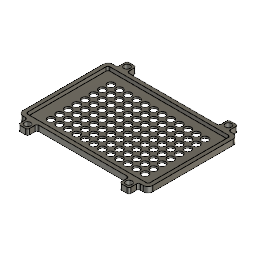
Plate_Adaptor_96 (Autodesk Fusion 360 design; units mm, degrees)
Autodesk Fusion 360 part; units mm, degrees
sketch "Sketch1" plane through (0, 0, 0) normal (0, 0, 1) x (1, 0, 0)
  line L0 (-68.38, 47.37) -> (68.38, 47.37)
  line L1 (68.38, 47.37) -> (68.38, -47.37)
  line L2 (68.38, -47.37) -> (-68.38, -47.37)
  line L3 (-68.38, -47.37) -> (-68.38, 47.37)
  line L4 (-68.38, 47.37) -> (68.38, -47.37) construction
  line L5 (68.38, 47.37) -> (-68.38, -47.37) construction
  line L6 (-58.38, 57.37) -> (-48.38, 57.37)
  line L7 (-48.38, 57.37) -> (-48.38, 47.37)
  line L8 (-48.38, 47.37) -> (-58.38, 47.37)
  line L9 (-58.38, 47.37) -> (-58.38, 57.37)
  line L10 (48.38, 57.37) -> (58.38, 57.37)
  line L11 (58.38, 57.37) -> (58.38, 47.37)
  line L12 (58.38, 47.37) -> (48.38, 47.37)
  line L13 (48.38, 47.37) -> (48.38, 57.37)
  line L14 (48.38, -47.37) -> (58.38, -47.37)
  line L15 (58.38, -47.37) -> (58.38, -57.37)
  line L16 (58.38, -57.37) -> (48.38, -57.37)
  line L17 (48.38, -57.37) -> (48.38, -47.37)
  line L18 (-58.38, -47.37) -> (-48.38, -47.37)
  line L19 (-48.38, -47.37) -> (-48.38, -57.37)
  line L20 (-48.38, -57.37) -> (-58.38, -57.37)
  line L21 (-58.38, -57.37) -> (-58.38, -47.37)
  line L22 (-49.5, 31.5) -> (49.5, 31.5)
  line L23 (49.5, 31.5) -> (49.5, -31.5)
  line L24 (49.5, -31.5) -> (-49.5, -31.5)
  line L25 (-49.5, -31.5) -> (-49.5, 31.5)
  line L26 (-49.5, 31.5) -> (49.5, -31.5) construction
  line L27 (49.5, 31.5) -> (-49.5, -31.5) construction
  circle A0 centre (-49.5, -31.5) radius 3.575
  circle A1 centre (-40.5, -31.5) radius 3.575
  circle A2 centre (-31.5, -31.5) radius 3.575
  circle A3 centre (-22.5, -31.5) radius 3.575
  circle A4 centre (-13.5, -31.5) radius 3.575
  circle A5 centre (-4.5, -31.5) radius 3.575
  circle A6 centre (4.5, -31.5) radius 3.575
  circle A7 centre (13.5, -31.5) radius 3.575
  circle A8 centre (22.5, -31.5) radius 3.575
  circle A9 centre (31.5, -31.5) radius 3.575
  circle A10 centre (40.5, -31.5) radius 3.575
  circle A11 centre (49.5, -31.5) radius 3.575
  circle A12 centre (-49.5, -22.5) radius 3.575
  circle A13 centre (-40.5, -22.5) radius 3.575
  circle A14 centre (-31.5, -22.5) radius 3.575
  circle A15 centre (-22.5, -22.5) radius 3.575
  circle A16 centre (-13.5, -22.5) radius 3.575
  circle A17 centre (-4.5, -22.5) radius 3.575
  circle A18 centre (4.5, -22.5) radius 3.575
  circle A19 centre (13.5, -22.5) radius 3.575
  circle A20 centre (22.5, -22.5) radius 3.575
  circle A21 centre (31.5, -22.5) radius 3.575
  circle A22 centre (40.5, -22.5) radius 3.575
  circle A23 centre (49.5, -22.5) radius 3.575
  circle A24 centre (-49.5, -13.5) radius 3.575
  circle A25 centre (-40.5, -13.5) radius 3.575
  circle A26 centre (-31.5, -13.5) radius 3.575
  circle A27 centre (-22.5, -13.5) radius 3.575
  circle A28 centre (-13.5, -13.5) radius 3.575
  circle A29 centre (-4.5, -13.5) radius 3.575
  circle A30 centre (4.5, -13.5) radius 3.575
  circle A31 centre (13.5, -13.5) radius 3.575
  circle A32 centre (22.5, -13.5) radius 3.575
  circle A33 centre (31.5, -13.5) radius 3.575
  circle A34 centre (40.5, -13.5) radius 3.575
  circle A35 centre (49.5, -13.5) radius 3.575
  circle A36 centre (-49.5, -4.5) radius 3.575
  circle A37 centre (-40.5, -4.5) radius 3.575
  circle A38 centre (-31.5, -4.5) radius 3.575
  circle A39 centre (-22.5, -4.5) radius 3.575
  circle A40 centre (-13.5, -4.5) radius 3.575
  circle A41 centre (-4.5, -4.5) radius 3.575
  circle A42 centre (4.5, -4.5) radius 3.575
  circle A43 centre (13.5, -4.5) radius 3.575
  circle A44 centre (22.5, -4.5) radius 3.575
  circle A45 centre (31.5, -4.5) radius 3.575
  circle A46 centre (40.5, -4.5) radius 3.575
  circle A47 centre (49.5, -4.5) radius 3.575
  circle A48 centre (-49.5, 4.5) radius 3.575
  circle A49 centre (-40.5, 4.5) radius 3.575
  circle A50 centre (-31.5, 4.5) radius 3.575
  circle A51 centre (-22.5, 4.5) radius 3.575
  circle A52 centre (-13.5, 4.5) radius 3.575
  circle A53 centre (-4.5, 4.5) radius 3.575
  circle A54 centre (4.5, 4.5) radius 3.575
  circle A55 centre (13.5, 4.5) radius 3.575
  circle A56 centre (22.5, 4.5) radius 3.575
  circle A57 centre (31.5, 4.5) radius 3.575
  circle A58 centre (40.5, 4.5) radius 3.575
  circle A59 centre (49.5, 4.5) radius 3.575
  circle A60 centre (-49.5, 13.5) radius 3.575
  circle A61 centre (-40.5, 13.5) radius 3.575
  circle A62 centre (-31.5, 13.5) radius 3.575
  circle A63 centre (-22.5, 13.5) radius 3.575
  circle A64 centre (-13.5, 13.5) radius 3.575
  circle A65 centre (-4.5, 13.5) radius 3.575
  circle A66 centre (4.5, 13.5) radius 3.575
  circle A67 centre (13.5, 13.5) radius 3.575
  circle A68 centre (22.5, 13.5) radius 3.575
  circle A69 centre (31.5, 13.5) radius 3.575
  circle A70 centre (40.5, 13.5) radius 3.575
  circle A71 centre (49.5, 13.5) radius 3.575
  circle A72 centre (-49.5, 22.5) radius 3.575
  circle A73 centre (-40.5, 22.5) radius 3.575
  circle A74 centre (-31.5, 22.5) radius 3.575
  circle A75 centre (-22.5, 22.5) radius 3.575
  circle A76 centre (-13.5, 22.5) radius 3.575
  circle A77 centre (-4.5, 22.5) radius 3.575
  circle A78 centre (4.5, 22.5) radius 3.575
  circle A79 centre (13.5, 22.5) radius 3.575
  circle A80 centre (22.5, 22.5) radius 3.575
  circle A81 centre (31.5, 22.5) radius 3.575
  circle A82 centre (40.5, 22.5) radius 3.575
  circle A83 centre (49.5, 22.5) radius 3.575
  circle A84 centre (-49.5, 31.5) radius 3.575
  circle A85 centre (-40.5, 31.5) radius 3.575
  circle A86 centre (-31.5, 31.5) radius 3.575
  circle A87 centre (-22.5, 31.5) radius 3.575
  circle A88 centre (-13.5, 31.5) radius 3.575
  circle A89 centre (-4.5, 31.5) radius 3.575
  circle A90 centre (4.5, 31.5) radius 3.575
  circle A91 centre (13.5, 31.5) radius 3.575
  circle A92 centre (22.5, 31.5) radius 3.575
  circle A93 centre (31.5, 31.5) radius 3.575
  circle A94 centre (40.5, 31.5) radius 3.575
  circle A95 centre (49.5, 31.5) radius 3.575
  point P0 (-57.3369, -42.2056)
  point P1 (-53.88, -84.89)
  dimension "d1" = 136.76
  dimension "d2" = 94.74
  dimension "d3" = 10
  dimension "d4" = 10
  dimension "d5" = 10
  dimension "d6" = 10
  dimension "d7" = 63
  dimension "d8" = 99
  dimension "d10" = 7.15
  dimension "d13" = 99
  dimension "d14" = 63
  constraint perpendicular L0 L1
  constraint parallel L0 L2
  constraint parallel L1 L3
  constraint horizontal L0
  constraint coincident L4 origin
  constraint coincident L5 origin
  constraint horizontal L6
  constraint vertical L7
  constraint horizontal L8
  constraint vertical L9
  constraint coincident L0 L7.end
  constraint horizontal L10
  constraint vertical L11
  constraint horizontal L12
  constraint vertical L13
  constraint horizontal L14
  constraint vertical L15
  constraint horizontal L16
  constraint vertical L17
  constraint horizontal L18
  constraint vertical L19
  constraint horizontal L20
  constraint vertical L21
  constraint perpendicular L22 L23
  constraint parallel L22 L24
  constraint parallel L23 L25
  constraint horizontal L22
  constraint coincident L26 origin
  constraint coincident L27 origin
  measures "d1" distance of L1 L3
  measures "d2" distance of L0.start L2.end
  measures "d3" distance of L6.start L6.end
  measures "d4" distance of L6.start L8.end
  measures "d5" distance of L10.start L10.end
  measures "d6" distance of L10.start L12.end
  measures "d7" distance of L22.end L23.end
  measures "d8" distance of L23.end L24.end
  measures "d10" diameter of A0
extrude "Extrude1" add sketch "Sketch1" along normal mid plane 6 contours L0 L1 L2 L3 L8 L12 L14 L18 | L0 L6 L7 L8 L9 | L2 L18 L19 L20 L21 | L0 L10 L11 L12 L13 | L2 L14 L15 L16 L17 | L22 L23 L24 L25 A0 A1 A2 A3 A4 A5 A6 A7 A8 A9 A10 A11 A12 A23 A24 A35 A36 A47 A48 A59 A60 A71 A72 A83 A84 A85 A86 A87 A88 A89 A90 A91 A92 A93 A94 A95
ref_plane "WorkPlane1" through (0, 0, 3) normal (0, 0, 1) x (1, 0, 0)
sketch "Sketch2" plane through (0, 0, 3) normal (0, 0, 1) x (1, 0, 0)
  line L0 (-64.38, 43.235) -> (64.38, 43.235)
  line L1 (64.38, 43.235) -> (64.38, -43.235)
  line L2 (64.38, -43.235) -> (-64.38, -43.235)
  line L3 (-64.38, -43.235) -> (-64.38, 43.235)
  line L4 (-64.38, 43.235) -> (64.38, -43.235) construction
  line L5 (64.38, 43.235) -> (-64.38, -43.235) construction
  dimension "d18" = 128.76
  dimension "d19" = 86.47
  constraint perpendicular L0 L1
  constraint parallel L0 L2
  constraint parallel L1 L3
  constraint horizontal L0
  constraint coincident L4 origin
  constraint coincident L5 origin
  measures "d18" distance of L1.end L2.end
  measures "d19" distance of L0.end L1.end
extrude "Extrude2" cut sketch "Sketch2" against normal blind 4
sketch "Sketch3" plane through (0, 0, 3) normal (0, 0, 1) x (-1, 0, 0)
  line L0 (-64.38, -43.235) -> (-64.38, 43.235)
  line L1 (-64.38, 43.235) -> (64.38, 43.235)
  line L2 (64.38, 43.235) -> (64.38, -43.235)
  line L3 (64.38, -43.235) -> (-64.38, -43.235)
  line L4 (58.38, 57.37) -> (48.38, 57.37)
  line L5 (48.38, 57.37) -> (48.38, 47.37)
  line L6 (48.38, 47.37) -> (-48.38, 47.37)
  line L7 (-48.38, 47.37) -> (-48.38, 57.37)
  line L8 (-48.38, 57.37) -> (-58.38, 57.37)
  line L9 (-58.38, 57.37) -> (-58.38, 47.37)
  line L10 (-58.38, 47.37) -> (-68.38, 47.37)
  line L11 (-68.38, 47.37) -> (-68.38, -47.37)
  line L12 (-68.38, -47.37) -> (-58.38, -47.37)
  line L13 (-58.38, -47.37) -> (-58.38, -57.37)
  line L14 (-58.38, -57.37) -> (-48.38, -57.37)
  line L15 (-48.38, -57.37) -> (-48.38, -47.37)
  line L16 (-48.38, -47.37) -> (48.38, -47.37)
  line L17 (48.38, -47.37) -> (48.38, -57.37)
  line L18 (48.38, -57.37) -> (58.38, -57.37)
  line L19 (58.38, -57.37) -> (58.38, -47.37)
  line L20 (58.38, -47.37) -> (68.38, -47.37)
  line L21 (68.38, -47.37) -> (68.38, 47.37)
  line L22 (68.38, 47.37) -> (58.38, 47.37)
  line L23 (58.38, 47.37) -> (58.38, 57.37)
  circle A0 centre (53.38, -52.37) radius 3.25
  circle A1 centre (-53.38, -52.3704) radius 3.25
  circle A2 centre (-53.38, 52.3703) radius 3.25
  circle A3 centre (53.38, 52.37) radius 3.25
  dimension "d22" = 6.5
  dimension "d23" = 6.5
  dimension "d24" = 6.5
  dimension "d25" = 6.5
  measures "d22" diameter of A0
  measures "d23" diameter of A1
  measures "d24" diameter of A2
  measures "d25" diameter of A3
extrude "Extrude3" cut sketch "Sketch3" against normal blind 6 contours A0 | A1 | A2 | A3
fillet "Fillet1" radius 5 4 edges at (68.38, -47.37, 0) (68.38, 47.37, 0) (-68.38, -47.37, 0) (-68.38, 47.37, 0)
fillet "Fillet2" radius 2 4 edges at (64.38, 43.235, 1) (-64.38, 43.235, 1) (-64.38, -43.235, 1) (64.38, -43.235, 1)
fillet "Fillet3" radius 2 16 edges at (48.38, 47.37, 0) (48.38, 57.37, 0) (58.38, 57.37, 0) (-58.38, 47.37, 0) (-58.38, 57.37, 0) (-48.38, 57.37, 0) (-48.38, 47.37, 0) (58.38, 47.37, 0) (58.38, -47.37, 0) (58.38, -57.37, 0) (48.38, -57.37, 0) (-48.38, -47.37, 0) (-48.38, -57.37, 0) (48.38, -47.37, 0) (-58.38, -47.37, 0) (-58.38, -57.37, 0)
